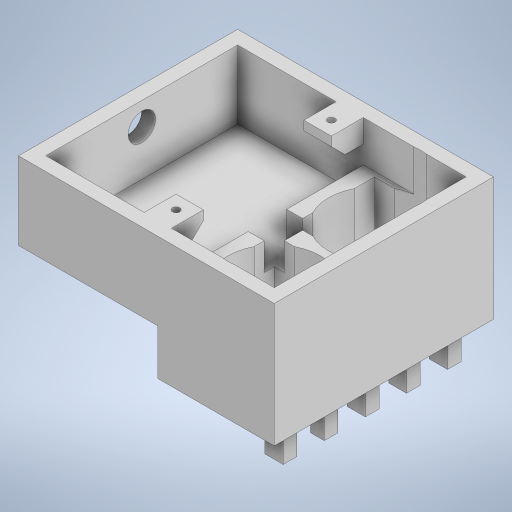
# Autodesk Inventor part: Suporte Eletroimã
Saved by Autodesk Inventor 2023 (Build 270158000, 158)
## iProperties
Created: 2023-03-07
Part Number: Suporte Eletroimã
Material: Genérico
Document SubType Name: Modeling
Designer: Inteli
Density: 1 g/cm^3
Appearance: Padrão
Author: Inteli
## iProperties of the stored document Suporte Eletroimã_3DPrint.ipt
Created: 2023-03-09
Part Number: Suporte Eletroimã_3DPrint
Material: Genérico
Document SubType Name: Modeling
Designer: Inteli
Density: 1 g/cm^3
Appearance: Padrão
Author: Inteli
Autodesk Inventor part; units mm, degrees
ref_plane "YZ Plane" through (0, 0, 0) normal (1, 0, 0) x (0, 1, 0)
ref_plane "XZ Plane" through (0, 0, 0) normal (0, 1, 0) x (-1, 0, 0)
ref_plane "XY Plane" through (0, 0, 0) normal (0, 0, 1) x (1, 0, 0)
sketch "Esboço1" plane through (0, 0, 0) normal (0, 1, 0) x (-1, 0, 0)
  circle A0 centre (0, 11) radius 10.1
  circle A1 centre (0, -11) radius 10.1
  line L0 (9, 2) -> (-9, 2)
  line L1 (-9, -2) -> (9, -2)
  line L2 (9, 20) -> (-9, 20)
  line L3 (-9, -20) -> (9, -20)
  line L4 (43, 24) -> (-13, 24)
  line L5 (-13, 24) -> (-13, -24)
  line L6 (-13, -24) -> (43, -24)
  line L7 (43, -24) -> (43, 24)
  line L8 (9, -20) -> (9, -2)
  line L9 (9, 2) -> (9, 20)
  line L10 (-9, 20) -> (-9, 2)
  line L11 (-9, -2) -> (-9, -20)
  point P0 (-9, 6.4163)
  point P1 (-9, 15.5837)
  point P2 (-4.5837, 20)
  point P3 (4.5837, 20)
  point P4 (9, 15.5837)
  point P5 (9, 6.4163)
  point P6 (4.5837, 2)
  point P7 (-4.5837, 2)
  point P8 (-9, -6.4163)
  point P9 (-4.5837, -2)
  point P10 (4.5837, -2)
  point P11 (9, -6.4163)
  point P12 (9, -15.5837)
  point P13 (4.5837, -20)
  point P14 (-4.5837, -20)
  point P15 (-9, -15.5837)
  point P16 (0, 0)
  point P17 (0, 21.1)
  point P18 (0, 21.1)
  point P19 (0, -21.1)
  point P20 (0, -21.1)
  dimension "d93" = 20.2
  dimension "d94" = 20.2
  dimension "d16" = 40
  dimension "d17" = 18
  dimension "d18" = 56
  dimension "d61" = 48
  dimension "d62" = 22
  constraints: 24 end point, 6 parallel, 3 coincident, 2 horizontal, 2 perpendicular, 1 vertical, 6 other
  measures "d16" distance of L3.start L2.end
  measures "d17" distance of L3.start L3.end
  measures "d18" distance of L6.end L5.end
  measures "d61" distance of L4.end L5.end
  measures "d62" distance of point (0, 11) point (0, -11)
extrude "Base Principal dos Imãs" add sketch "Esboço1" along normal blind 25
sketch "Esboço9" plane through (0, 0, 0) normal (0, -1, 0) x (1, 0, 0)
  line L0 (-43, 24) -> (13, 24) projected
  line L1 (13, -24) -> (-43, -24) projected
  line L2 (13, 24) -> (-43, 24)
  line L3 (-43, 24) -> (-43, -24)
  line L4 (-43, -24) -> (13, -24)
  line L5 (13, -24) -> (13, 24)
  point P0 (0, 0)
  point P1 (-43, 24)
  point P2 (13, -24)
  constraints: 8 end point, 2 parallel, 1 horizontal, 1 perpendicular
extrude "Fundo" add sketch "Esboço9" along normal blind 2
sketch "Esboço13" plane through (0, 25, 0) normal (0, 1, 0) x (1, 0, 0)
  line L0 (10, 21) -> (-40, 21)
  line L1 (-40, 21) -> (-40, -21)
  line L2 (-40, -21) -> (10, -21)
  line L3 (10, -21) -> (10, 21)
  line L4 (10, 21) -> (-40, -21) construction
  line L5 (-40, 21) -> (10, -21) construction
  line L6 (13, 24) -> (-43, 24) projected
  point P0 (0, 0)
  point P1 (0, 0)
  point P2 (25, 0)
  point P3 (10, 0)
  dimension "d84" = 50
  constraints: 12 end point, 1 coincident, 1 horizontal, 1 vertical
  measures "d84" distance of L2.end L1.end
extrude "PCB / Tampa" cut sketch "Esboço13" against normal blind 9
sketch "Esboço14" plane through (0, 25, 0) normal (0, 1, 0) x (1, 0, 0)
  line L0 (-9, -2) -> (-4.5837, -2) projected
  line L1 (-6.7918, -2) -> (-9, -4.2082)
  line L2 (-9, -6.4163) -> (-9, -2) projected
  line L3 (-6.7918, -2) -> (-6.7918, 2)
  line L4 (-9, 2) -> (-4.5837, 2) projected
  line L5 (-9, 2) -> (-9, 6.4163) projected
  line L6 (-9, 4.2082) -> (-6.7918, 2)
  line L7 (-9, -4.2082) -> (-12.5, -4.2082)
  line L8 (-12.5, -4.2082) -> (-12.5, 4.2082)
  line L9 (-12.5, 4.2082) -> (-9, 4.2082)
  point P0 (0, 0)
  dimension "d183" = 3.5
  constraints: 12 end point, 4 midpoint, 3 perpendicular, 1 horizontal
  measures "d183" distance of L1.end L7.end
extrude "Espaço Fio (Validar)" cut sketch "Esboço14" against normal blind 15
sketch "Esboço16" plane through (0, -2, 0) normal (0, -1, 0) x (1, 0, 0)
  line L0 (13, 24) -> (-43, 24) projected
  line L1 (-43, -24) -> (13, -24) projected
  line L2 (13, -24) -> (13, 24) projected
  line L3 (10.5, 19.552) -> (6.5, 19.552)
  line L4 (6.5, 19.552) -> (6.5, 16.5634)
  line L5 (6.5, 16.5634) -> (10.5, 16.5634)
  line L6 (10.5, 16.5634) -> (10.5, 19.552)
  line L7 (10.5, 19.552) -> (6.5, 16.5634) construction
  line L8 (6.5, 19.552) -> (10.5, 16.5634) construction
  line L9 (10.5, 10.552) -> (6.5, 10.552)
  line L10 (6.5, 10.552) -> (6.5, 7.5634)
  line L11 (6.5, 7.5634) -> (10.5, 7.5634)
  line L12 (10.5, 7.5634) -> (10.5, 10.552)
  line L13 (10.5, 10.552) -> (6.5, 7.5634) construction
  line L14 (6.5, 10.552) -> (10.5, 7.5634) construction
  line L15 (10.5, 1.552) -> (6.5, 1.552)
  line L16 (6.5, 1.552) -> (6.5, -1.4366)
  line L17 (6.5, -1.4366) -> (10.5, -1.4366)
  line L18 (10.5, -1.4366) -> (10.5, 1.552)
  line L19 (10.5, 1.552) -> (6.5, -1.4366) construction
  line L20 (6.5, 1.552) -> (10.5, -1.4366) construction
  line L21 (10.5, -7.448) -> (6.5, -7.448)
  line L22 (6.5, -7.448) -> (6.5, -10.4366)
  line L23 (6.5, -10.4366) -> (10.5, -10.4366)
  line L24 (10.5, -10.4366) -> (10.5, -7.448)
  line L25 (10.5, -7.448) -> (6.5, -10.4366) construction
  line L26 (6.5, -7.448) -> (10.5, -10.4366) construction
  line L27 (10.5, -16.448) -> (6.5, -16.448)
  line L28 (6.5, -16.448) -> (6.5, -19.4366)
  line L29 (6.5, -19.4366) -> (10.5, -19.4366)
  line L30 (10.5, -19.4366) -> (10.5, -16.448)
  line L31 (10.5, -16.448) -> (6.5, -19.4366) construction
  line L32 (6.5, -16.448) -> (10.5, -19.4366) construction
  point P0 (0, 0)
  point P1 (8.5, 18.0577)
  point P2 (8.5, 9.0577)
  point P3 (8.5, 0.0577)
  point P4 (8.5, -8.9423)
  point P5 (8.5, -17.9423)
  dimension "d132" = 9
  dimension "d144" = 9
  dimension "d187" = 4
  dimension "d192" = 2.5
  constraints: 60 end point, 2 midpoint, 2 parallel, 2 vertical, 1 horizontal, 1 perpendicular, 44 other
  measures "d144" distance of L3.start L9.start
  measures "d187" distance of L10.end L11.end
  measures "d192" distance between parallel lines of L2 L6
sketch "Esboço17" plane through (-43, 25, -24) normal (-1, 0, 0) x (0, 0, 1)
  line L0 (0, -27) -> (0, 0) projected
  line L1 (48, -27) -> (48, 0) projected
  line L2 (0, 0) -> (48, 0)
  line L3 (48, 0) -> (48, -3)
  line L4 (48, -3) -> (0, -3)
  line L5 (0, -3) -> (0, 0)
  point P0 (24, -25)
  point P1 (0, -3)
  dimension "d109" = 3
  constraints: 8 end point, 2 parallel, 1 horizontal, 1 perpendicular, 1 point on line
  measures "d109" distance of L2.end L3.end
sketch "Esboço19" plane through (-43, -2, -24) normal (-1, 0, 0) x (0, 0, 1)
  line L0 (48, 0) -> (0, 0) projected
  line L1 (17.5, 20) -> (28.5, 20)
  line L2 (28.5, 20) -> (28.5, 12)
  line L3 (28.5, 12) -> (17.5, 12)
  line L4 (17.5, 12) -> (17.5, 20)
  line L5 (0, 24) -> (46, 24) projected
  point P0 (24, 2)
  dimension "d123" = 11
  dimension "d124" = 8
  constraints: 8 end point, 2 parallel, 1 horizontal, 1 perpendicular
  measures "d123" distance of L2.end L3.end
  measures "d124" distance of L1.end L2.end
extrude "Extrusão19" add sketch "Esboço16" along normal blind 7
fillet "Arredondamento da face2" radius 1 1 edges at (6.5, -2, 18.0577)
fillet "Arredondamento da face3" radius 1 2 edges at (6, -2, 19.552) (8.5, -2, 19.552)
fillet "Arredondamento da face4" radius 1 2 edges at (10.5, -2, 20.052) (10.5, -2, 18.0577)
fillet "Arredondamento da face5" radius 1 3 edges at (11, -2, 16.5634) (8.5, -2, 16.5634) (6, -2, 16.5634)
fillet "Arredondamento da face6" radius 1 1 edges at (10.5, -2, 9.0577)
fillet "Arredondamento da face7" radius 1 2 edges at (11, -2, 10.552) (8.5, -2, 10.552)
fillet "Arredondamento da face8" radius 1 1 edges at (6.5, -2, 9.5577)
fillet "Arredondamento da face9" radius 1 2 edges at (6, -2, 7.5634) (9, -2, 7.5634)
fillet "Arredondamento da face10" radius 1 1 edges at (6.5, -2, 0.0577)
fillet "Arredondamento da face11" radius 1 2 edges at (6, -2, -1.4366) (8.5, -2, -1.4366)
fillet "Arredondamento da face12" radius 1 2 edges at (8.5, -2, 1.552) (6, -2, 1.552)
fillet "Arredondamento da face13" radius 1 3 edges at (10.5, -2, 2.052) (10.5, -2, 0.0577) (10.5, -2, -1.9366)
fillet "Arredondamento da face14" radius 1 1 edges at (10.5, -2, -8.9423)
fillet "Arredondamento da face15" radius 1 2 edges at (11, -2, -7.448) (8.5, -2, -7.448)
fillet "Arredondamento da face16" radius 1 2 edges at (6.5, -2, -6.948) (6.5, -2, -8.9423)
fillet "Arredondamento da face17" radius 1 3 edges at (11, -2, -10.4366) (8.5, -2, -10.4366) (6, -2, -10.4366)
fillet "Arredondamento da face18" radius 1 1 edges at (8.5, -2, -19.4366)
fillet "Arredondamento da face19" radius 1 2 edges at (10.5, -2, -19.9366) (10.5, -2, -17.9423)
fillet "Arredondamento da face20" radius 1 2 edges at (6.5, -2, -19.9366) (6.5, -2, -17.9423)
fillet "Arredondamento da face21" radius 1 3 edges at (6, -2, -16.448) (8.5, -2, -16.448) (11, -2, -16.448)
sketch "Esboço21" plane through (0, -2, 0) normal (0, -1, 0) x (1, 0, 0)
  arc A0 (-9, -6.4163) -> (-9, -15.5837) centre (0, -11) ccw projected
  line L0 (13, 24) -> (-43, 24) projected
  line L1 (-43, 24) -> (-43, -24)
  line L2 (-43, -24) -> (-12.5, -24)
  line L3 (-12.5, -24) -> (-12.5, -11)
  line L4 (-12.5, -11) -> (-12.5, 24)
  line L5 (-43, -24) -> (13, -24) projected
  line L6 (-12.5, 24) -> (-43, 24)
  line L7 (-43, 24) -> (-43, -24) projected
  point P0 (0, 0)
  constraints: 10 end point, 2 point on line, 1 collinear, 1 perpendicular
extrude "Rebaixo Externo" cut sketch "Esboço21" against normal blind 10
sketch "Esboço22" plane through (0, 16, 0) normal (0, 1, 0) x (1, 0, 0)
  line L0 (-12.5, -24) -> (-12.5, 24) projected
  line L1 (-40, 21) -> (-1.4177, 21) projected
  line L2 (-12.5, 21) -> (-40, 21)
  line L3 (-40, -21) -> (-40, 21) projected
  line L4 (-40, 21) -> (-40, -21)
  line L5 (-40, -21) -> (-12.5, -21)
  line L6 (-12.5, -21) -> (-12.5, 21)
  point P0 (0, 0)
  point P1 (-12.5, 21)
  constraints: 8 end point, 2 collinear, 2 perpendicular, 1 point on line
extrude "Espaço Fios" cut sketch "Esboço22" against normal blind 6
sketch "Esboço23" plane through (-40, 25, 21) normal (1, 0, 0) x (0, 0, -1)
  circle A0 centre (21, -5) radius 3
  circle A1 centre (21, -5) radius 3
  dimension "d206" = 6
  constraints: 2 centre point, 1 coincident
  measures "d206" diameter of A0
extrude "Furo LED" cut sketch "Esboço23" against normal up to surface (3 mm away)
sketch "Esboço24" plane through (0, 0, 0) normal (0, 1, 0) x (1, 0, 0)
  arc A0 (-4.5837, -20) -> (4.5837, -20) centre (0, -11) ccw projected
  circle A1 centre (0, -11) radius 7.5
  arc A2 (4.5837, 20) -> (-4.5837, 20) centre (0, 11) ccw projected
  circle A3 centre (0, 11) radius 7.5
  point P0 (0, 0)
  dimension "d188" = 15
  dimension "d189" = 15
  constraints: 2 centre point, 2 coincident
  measures "d188" diameter of A1
  measures "d189" diameter of A3
extrude "Extrusão23" cut sketch "Esboço24" against normal up to surface (9 mm away)
sketch "Esboço25" plane through (0, 25, 0) normal (0, 1, 0) x (1, 0, 0)
  line L0 (-12.5, 21) -> (-18.5, 21)
  line L1 (-18.5, 21) -> (-18.5, 14)
  line L2 (-18.5, 14) -> (-12.5, 14)
  line L3 (-12.5, 14) -> (-12.5, 21)
  circle A0 centre (-15.5, 17) radius 0.8
  line L4 (-12.5, -24) -> (-12.5, 24) projected
  line L5 (-12.5, -21) -> (-18.5, -21)
  line L6 (-18.5, -21) -> (-18.5, -14)
  line L7 (-18.5, -14) -> (-12.5, -14)
  line L8 (-12.5, -14) -> (-12.5, -21)
  circle A1 centre (-15.5, -17) radius 0.8
  point P0 (0, 0)
  point P1 (-12.5, -14)
  dimension "d193" = 6
  dimension "d194" = 7
  dimension "d195" = 1.6
  dimension "d196" = 3
  dimension "d197" = 3
  dimension "d203" = 7
  dimension "d204" = 3
  dimension "d205" = 6
  constraints: 16 end point, 2 centre point, 2 parallel, 1 horizontal, 1 perpendicular
  measures "d193" distance of L2.end L1.end
  measures "d194" distance of L1.end L0.end
  measures "d195" diameter of A0
  measures "d196" distance from line of L1 A0.centre
  measures "d197" distance from line of A0.centre L2
  measures "d203" distance of L5.end L6.end
  measures "d204" distance from line of L7 A1.centre
  measures "d205" distance of L6.end L7.end
extrude "Extrusão24" add sketch "Esboço25" against normal blind 5
chamfer "Chanfro2" distance 3 angle 45 2 edges at (-15.5, 20, -14) (-15.5, 20, 14)
